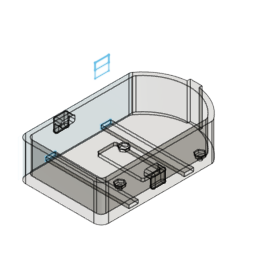
RyobiBatteryTank (Autodesk Fusion 360 design; units mm, degrees)
Autodesk Fusion 360 part; units mm, degrees
sketch "Sketch1" plane through (0, 0, 0) normal (0, 0, 1) x (1, 0, 0)
  line L0 (0, 0) -> (80, 0)
  line L1 (80, 0) -> (80, 135) construction
  line L2 (0, 135) -> (0, 0) construction
  line L3 (0, 135) -> (80, 135) construction
  line L4 (80, 135) -> (80, 115) construction
  line L5 (80, 115) -> (0, 115) construction
  arc A0 (80, 115) -> (0, 115) centre (40, 85) ccw
  line L6 (0, 0) -> (0, 115)
  line L7 (80, 115) -> (80, 0)
  line L8 (-5, -5) -> (85, -5)
  line L9 (85, 116.6228) -> (85, -5)
  arc A1 (85, 116.6228) -> (-5, 116.6228) centre (40, 85) ccw
  line L10 (-5, -5) -> (-5, 116.6228)
  line L11 (33.5, 143) -> (46.5, 143)
  line L12 (46.5, 143) -> (46.5, 135)
  line L13 (46.5, 135) -> (33.5, 135)
  line L14 (33.5, 135) -> (33.5, 143)
  circle A2 centre (74.4902, 112.6066) radius 2
  circle A3 centre (74.4902, 112.6066) radius 4 construction
  line L15 (78.4402, 114.8871) -> (74.4902, 117.1677)
  line L16 (74.4902, 117.1677) -> (70.5402, 114.8871)
  line L17 (70.5402, 114.8871) -> (70.5402, 110.3261)
  line L18 (70.5402, 110.3261) -> (74.4902, 108.0455)
  line L19 (74.4902, 108.0455) -> (78.4402, 110.3261)
  line L20 (78.4402, 110.3261) -> (78.4402, 114.8871)
  line L21 (26.3395, 82.5602) -> (22.5205, 80.0545)
  circle A4 centre (26.6, 78) radius 4 construction
  circle A5 centre (26.6, 78) radius 2
  line L22 (26.8605, 73.4398) -> (30.6795, 75.9455)
  line L23 (22.781, 75.4943) -> (26.8605, 73.4398)
  line L24 (22.5205, 80.0545) -> (22.781, 75.4943)
  line L25 (30.6795, 75.9455) -> (30.419, 80.5057)
  line L26 (30.419, 80.5057) -> (26.3395, 82.5602)
  line L27 (58.9665, 36.8424) -> (62.8002, 39.3174)
  line L28 (54.9063, 38.9251) -> (58.9665, 36.8424)
  line L29 (62.5737, 43.8749) -> (58.5135, 45.9576)
  line L30 (62.8002, 39.3174) -> (62.5737, 43.8749)
  circle A6 centre (58.74, 41.4) radius 4 construction
  line L31 (58.5135, 45.9576) -> (54.6798, 43.4826)
  line L32 (54.6798, 43.4826) -> (54.9063, 38.9251)
  circle A7 centre (58.74, 41.4) radius 2
  line L33 (85, -5) -> (58.74, -5) construction
  line L34 (58.74, -5) -> (58.74, 41.4) construction
  line L35 (58.74, 41.4) -> (85, 41.4) construction
  line L36 (85, 41.4) -> (85, -5) construction
  line L37 (-5, 78) -> (26.6, 78) construction
  line L38 (26.6, 78) -> (26.6, -5) construction
  line L39 (26.6, -5) -> (-5, -5) construction
  line L40 (-5, -5) -> (-5, 78) construction
  circle A8 centre (167.6575, 118.9529) radius 2.1
  line L41 (65, 60.1571) -> (15, 60.1571)
  line L42 (15, 60.1571) -> (15, 80.1571)
  line L43 (15, 80.1571) -> (65, 80.1571)
  line L44 (65, 80.1571) -> (65, 60.1571)
  line L45 (15, 80.1571) -> (65, 60.1571) construction
  line L46 (15, 60.1571) -> (65, 80.1571) construction
  line L47 (40, 70.1571) -> (40, 159.8429) construction
  point P0 (74.4902, 112.6066)
  point P1 (26.6, 78)
  point P2 (61.8152, 38.8847)
  point P3 (58.74, 41.4)
  dimension "d1" = 80
  dimension "d2" = 135
  dimension "d3" = 20
  dimension "d4" = -5
  dimension "d9" = 13
  dimension "d10" = 8
  dimension "d31" = 4
  dimension "d32" = 8
  dimension "d35" = 4
  dimension "d36" = 8
  dimension "d42" = 4
  dimension "d43" = 8
  dimension "d44" = 26.26
  dimension "d45" = 46.4
  dimension "d46" = 31.6
  dimension "d47" = 83
  dimension "d48" = 4.2
  dimension "d49" = 50
  dimension "d50" = 20
  constraint horizontal L0
  constraint vertical L1
  constraint vertical L2
  constraint coincident L0.start L2.end
  constraint horizontal L3
  constraint vertical L4
  constraint horizontal L5
  constraint tangent L3 A0
  constraint perpendicular L5 L6
  constraint perpendicular L0 L7
  constraint horizontal L11
  constraint vertical L12
  constraint horizontal L13
  constraint vertical L14
  constraint midpoint A0 L13
  constraint concentric A2 A3
  constraint coincident P0 A2.centre
  constraint concentric A4 A5
  constraint coincident P1 A4.centre
  constraint concentric A6 A7
  constraint coincident P3 A6.centre
  constraint horizontal L33
  constraint vertical L34
  constraint horizontal L35
  constraint vertical L36
  constraint coincident L8.end L9.end
  constraint horizontal L37
  constraint vertical L38
  constraint horizontal L39
  constraint vertical L40
  constraint coincident L8.start L10.start
  constraint horizontal L41
  constraint vertical L42
  constraint horizontal L43
  constraint vertical L44
  constraint midpoint L45 L47.start
  constraint perpendicular L43 L47
  constraint midpoint L5 L47
  measures "d1" distance of L0.start L0.end
  measures "d2" distance of L0.start L2.start
  measures "d3" distance of L2.start L5.end
  measures "d9" distance of L11.start L11.end
  measures "d10" distance of L11.start L13.end
  measures "d31" diameter of A2
  measures "d32" diameter of A3
  measures "d35" diameter of A5
  measures "d36" diameter of A4
  measures "d42" diameter of A7
  measures "d43" diameter of A6
  measures "d44" distance of L8.end L33.end
  measures "d45" distance of L8.end L35.end
  measures "d46" distance of L37.start P1
  measures "d47" distance of L37.start L8.start
  measures "d48" diameter of A8
  measures "d49" distance of L41.start L41.end
  measures "d50" distance of L41.start L43.end
extrude "Floor" add sketch "Sketch1" along normal blind 6 contours L0 A0 L6 L7 | L8 L9 A1 L10 L12 L13 L14 | A1 L12 L13 L14 | A2 | L15 L16 L17 L18 L19 L20 | L21 L25 L26 L43 | L21 L22 L23 L24 L25 L43 | L21 L22 L23 L24 L25 L41 L42 L43 L44 | A5 | L27 L28 L29 L30 L31 L32 | A7 makes body 1
extrude "Sides" add sketch "Sketch1" along normal blind 40 contours L8 L9 A1 L10 L12 L13 L14 | A1 L12 L13 L14 bodies 1
extrude "Extrude3" add sketch "Sketch1" along normal blind 40 contours A1 L12 L13 L14 | A1 L11 L12 L14 bodies 1
sketch "Sketch3" plane through (-5, 0, 0) normal (-1, 0, 0) x (0, -1, 0)
  line L0 (-116.6228, 0) -> (5, 0)
  line L1 (5, 0) -> (5, 40)
  line L2 (5, 40) -> (-116.6228, 40)
  line L3 (-116.6228, 40) -> (-116.6228, 0)
  line L4 (-95.0874, 6.3184) -> (-85.0874, 6.3184)
  line L5 (-85.0874, 6.3184) -> (-85.0874, 2.8184)
  line L6 (-85.0874, 2.8184) -> (-95.0874, 2.8184)
  line L7 (-95.0874, 2.8184) -> (-95.0874, 6.3184)
  line L8 (-35.0874, 2.8184) -> (-35.0874, 6.3184)
  line L9 (-25.0874, 6.3184) -> (-25.0874, 2.8184)
  line L10 (-35.0874, 6.3184) -> (-25.0874, 6.3184)
  line L11 (-25.0874, 2.8184) -> (-35.0874, 2.8184)
  line L12 (-93.2742, 68.1482) -> (-78.2742, 68.1482)
  line L13 (-78.2742, 68.1482) -> (-78.2742, 53.1482)
  line L14 (-78.2742, 53.1482) -> (-93.2742, 53.1482)
  line L15 (-93.2742, 53.1482) -> (-93.2742, 68.1482)
  line L16 (-93.2742, 68.1482) -> (-78.2742, 68.1482)
  line L17 (-78.2742, 68.1482) -> (-78.2742, 61.1482)
  line L18 (-78.2742, 61.1482) -> (-93.2742, 61.1482)
  line L19 (-93.2742, 61.1482) -> (-93.2742, 68.1482)
  dimension "d25" = 10
  dimension "d26" = 3.5
  dimension "d27" = 10
  dimension "d28" = 3.5
  dimension "d64" = 15
  dimension "d65" = 15
  dimension "d66" = 7
  constraint horizontal L4
  constraint vertical L5
  constraint horizontal L6
  constraint vertical L7
  constraint horizontal L10
  constraint vertical L9
  constraint horizontal L11
  constraint vertical L8
  constraint horizontal L12
  constraint vertical L13
  constraint horizontal L14
  constraint vertical L15
  constraint horizontal L16
  constraint vertical L17
  constraint horizontal L18
  constraint vertical L19
  measures "d25" distance of L4.start L4.end
  measures "d26" distance of L4.start L6.end
  measures "d27" distance of L9.start L8.end
  measures "d28" distance of L8.start L8.end
  measures "d64" distance of L12.start L12.end
  measures "d65" distance of L12.start L14.end
  measures "d66" distance of L12.start L18.end
extrude "CutSlotsOnBottom" cut sketch "Sketch3" against normal blind 100 contours L4 L5 L6 L7 | L8 L9 L10 L11 bodies 1
extrude "Extrude7" cut sketch "Sketch1" along normal blind 6 contours A2 | A5 | A7 bodies 1
extrude "Extrude8" cut sketch "Sketch1" along normal blind 2.9 from surface at 3.1 contours L15 L16 L17 L18 L19 L20 | L21 L25 L26 L43 | L21 L22 L23 L24 L25 L43 | L27 L28 L29 L30 L31 L32 bodies 1
extrude "Extrude9" cut sketch "Sketch1" along normal blind 3.2 contours L21 L22 L23 L24 L25 L43 | L21 L22 L23 L24 L25 L41 L42 L43 L44 | A5 bodies 1
fillet "Fillet1" radius 2 4 edges at (15, 60.1571, 1.6) (65, 60.1571, 1.6) (65, 80.1571, 1.6) (15, 80.1571, 1.6) on bodies 1
fillet "Fillet2" radius 5 2 edges at (0, 0, 23) (80, 0, 23) on bodies 1
fillet "Fillet3" radius 8 2 edges at (85, -5, 20) (-5, -5, 20) on bodies 1
fillet "Fillet4" radius 5 2 edges at (0, 115, 23) (80, 115, 23) on bodies 1
fillet "Fillet5" radius 5 2 edges at (85, 116.6228, 20) (-5, 116.6228, 20) on bodies 1
chamfer "Chamfer1" distance 0.5 angle 45 18 edges at (24.8207, 74.4671, 6) (22.6508, 77.7744, 6) (24.43, 81.3073, 6) (28.3793, 81.5329, 6) (30.5492, 78.2256, 6) (28.77, 74.6927, 6) (54.793, 41.2039, 6) (56.5966, 44.7201, 6) (60.5436, 44.9163, 6) (56.9364, 37.8837, 6) (60.8834, 38.0799, 6) (62.687, 41.5961, 6) (70.5402, 112.6066, 6) (72.5152, 116.0274, 6) (76.4652, 116.0274, 6) (78.4402, 112.6066, 6) (76.4652, 109.1858, 6) (72.5152, 109.1858, 6) on bodies 1
extrude "Extrude10" add sketch "Sketch3" along normal blind 10 separate body contours L12 L13 L15 L16 L17 L18 L19 makes body 2
extrude "Extrude11" add sketch "Sketch3" along normal blind 5 contours L13 L14 L15 L18 bodies 2
fillet "Fillet6" radius 2 12 edges at (-5, 93.2742, 60.6482) (-5, 85.7742, 68.1482) (-5, 78.2742, 60.6482) (-5, 85.7742, 53.1482) (-10, 93.2742, 68.1482) (-10, 78.2742, 68.1482) (-12.5, 93.2742, 61.1482) (-10, 93.2742, 57.1482) (-7.5, 93.2742, 53.1482) (-7.5, 78.2742, 53.1482) (-12.5, 78.2742, 61.1482) (-10, 78.2742, 57.1482) on bodies 2
move_body "Move1" bodies 2 to x (1, 0, 0) y (0, 1, 0) z (0, 0, 1) at (100.1268, -36.7132, 0)
copy_body "CopyPasteBodies1" bodies 2 makes body 3
move_body "Move2" bodies 3 to x (-1, 0, 0) y (0, -1, 0) z (0, 0, 1) at (79.9787, 98.122, 0)
move_body "Move3" bodies 3 2 to x (1, 0, 0) y (0, 1, 0) z (0, 0, 1) at (0, 0, -37.2216)
fillet "Fillet7" radius 2 6 edges at (90.7126, 55.9752, 16.5124) (90.1268, 49.061, 15.9266) (90.7126, 42.1468, 16.5124) (-10.7339, 42.1468, 16.5124) (-10.1481, 49.061, 15.9266) (-10.7339, 55.9752, 16.5124) on bodies 2 3
move_body "Move4" bodies 3 to x (1, 0, 0) y (0, 1, 0) z (0, 0, 1) at (0.3239, 0, 0)
move_body "Move5" bodies 2 to x (1, 0, 0) y (0, 1, 0) z (0, 0, 1) at (-0.2944, 0, 0)
combine "Combine1" operation add target body 1 tool bodies 3 2
